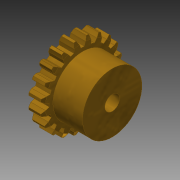
# Autodesk Inventor part: Zahnrad Messing z20
Saved by Autodesk Inventor 2019.4 (Build 234330000, 330)
## iProperties
Category: PARTsolutions
Company: MAEDLER
Created: 2018-08-20
Part Number: Zahnrad Messing z20
Material: Messing, weicher Gelbton, geschweißt
Catalog Web Link: www.cadenas.de
Description: Stzr Messing Ms58-Spur Gears, Brass, Helical Tooth Right Hand, with one-sided hub
Vendor: MAEDLER
Document SubType Name: Modeling
Designer: psadmin
Manufacturer: MAEDLER
Mass: 2.8 g
Surface Area: 3.98913 cm^2
Volume: 0.336189 cm^3
Density: 8.32866 g/cm^3
Appearance: Schweißnaht - Messing
PSOL_IDENT_0: {$CADENAS_DATA\23d-libs\maedler\antriebselemente\stirnzahnraeder\stirnzahnraeder_messing\stzr_messin
PSOL_IDENT_1: g_ms58.prj},204 {VTYP=3D},{NB=Stzr Messing Ms58 26102000},{LINA=Stzr Messing Ms58 26102000},{NN=Stzr
PSOL_IDENT_2: Messing Ms58},{DATE=03.08.2018 09:08:56},{GEOMDATE=26.07.2018 09:15:44},{VERSION=},{LINEID=270},{WB
PSOL_IDENT_3: VAR=},{WBNUMERIC=}  {NB=Stzr Messing Ms58 26102000},{LINA=Stzr Messing Ms58 26102000},{KT=DUMMY},{AR
PSOL_IDENT_4: TNR=26102000},{WST=Messing (Ms58)},{M=0.5},{Z=20},{PDF=PDF Katalogseite},{B1=2.0},{DA=11.00},{D=10.0
PSOL_IDENT_5: 0},{NL=4},{ND=8},{B=2.00},{MD=1.2},{GEW=2.800}
NN: Stzr Messing Ms58
NT: Spur Gears, Brass, Helical Tooth Right Hand, with one-sided hub
NB: Stzr Messing Ms58 26102000
NBSYN: Stzr Messing Ms58 $ARTNR.
LINA: Stzr Messing Ms58 26102000
ARTNR: 26102000
WST: Messing (Ms58)
M: 0.5
Z: 20
PDF: PDF Katalogseite
B1: 2
DA: 11
D: 10
NL: 4
ND: 8
B: 2
MD: 1.2
GEW: 2.8
SUPPLIER: MAEDLER
ARTICLENO: Stzr Messing Ms58 26102000
BOMINFO: Stzr Messing Ms58 26102000
CREATOR: CADENAS GmbH
Title: Stzr Messing Ms58 26102000
Author: Cadenas PARTsolutions
Comments: Spur Gears, Brass, Helical Tooth Right Hand, with one-sided hub
Autodesk Inventor part; units mm, degrees
ref_plane "YZ Plane" through (0, 0, 0) normal (1, 0, 0) x (0, 1, 0)
ref_plane "XZ Plane" through (0, 0, 0) normal (0, 1, 0) x (-1, 0, 0)
ref_plane "XY Plane" through (0, 0, 0) normal (0, 0, 1) x (1, 0, 0)
sketch "Skizze_1" plane through (0, 0, 0) normal (0, 0, 1) x (1, 0, 0)
  line L0 (6, 0) -> (0, 0)
  line L1 (0, 1) -> (6, 1)
  line L2 (6, 1) -> (6, 4)
  line L3 (6, 4) -> (2, 4)
  line L4 (2, 4) -> (2, 5)
  line L5 (2, 5) -> (1, 7.7475)
  line L6 (1, 7.7475) -> (0, 5)
  line L7 (0, 5) -> (0, 1)
  constraints: 16 end point
revolve "Revolution1" add sketch "Skizze_1" angle 360 about axis through (6, 0, 0) along (1, 0, 0)
sketch "Skizze_2" plane through (2, 0, 0) normal (1, 0, 0) x (0, 0, -1)
  circle A0 centre (0, 0) radius 16.5
  arc A1 (-5.4559, -0.6954) -> (-5.4037, -1.0246) centre (0, 0) ccw
  line L0 (-5.4037, -1.0246) -> (-4.8668, -1.1465)
  line L1 (-4.8668, -1.1465) -> (-4.3467, -1.1647)
  arc A2 (-4.3467, -1.1647) -> (-4.2011, -1.6127) centre (0, 0) ccw
  line L2 (-4.2011, -1.6127) -> (-4.6112, -1.9331)
  line L3 (-4.6112, -1.9331) -> (-4.974, -2.3473)
  arc A3 (-4.974, -2.3473) -> (-4.8226, -2.6443) centre (0, 0) ccw
  line L4 (-4.8226, -2.6443) -> (-4.2743, -2.5943)
  line L5 (-4.2743, -2.5943) -> (-3.774, -2.4509)
  arc A4 (-3.774, -2.4509) -> (-3.4972, -2.8319) centre (0, 0) ccw
  line L6 (-3.4972, -2.8319) -> (-3.7882, -3.2634)
  line L7 (-3.7882, -3.2634) -> (-4.0052, -3.7695)
  arc A5 (-4.0052, -3.7695) -> (-3.7695, -4.0052) centre (0, 0) ccw
  line L8 (-3.7695, -4.0052) -> (-3.2634, -3.7882)
  line L9 (-3.2634, -3.7882) -> (-2.8319, -3.4972)
  arc A6 (-2.8319, -3.4972) -> (-2.4509, -3.774) centre (0, 0) ccw
  line L10 (-2.4509, -3.774) -> (-2.5943, -4.2743)
  line L11 (-2.5943, -4.2743) -> (-2.6443, -4.8226)
  arc A7 (-2.6443, -4.8226) -> (-2.3473, -4.974) centre (0, 0) ccw
  line L12 (-2.3473, -4.974) -> (-1.9331, -4.6112)
  line L13 (-1.9331, -4.6112) -> (-1.6127, -4.2011)
  arc A8 (-1.6127, -4.2011) -> (-1.1647, -4.3467) centre (0, 0) ccw
  line L14 (-1.1647, -4.3467) -> (-1.1465, -4.8668)
  line L15 (-1.1465, -4.8668) -> (-1.0246, -5.4037)
  arc A9 (-1.0246, -5.4037) -> (-0.6954, -5.4559) centre (0, 0) ccw
  line L16 (-0.6954, -5.4559) -> (-0.4135, -4.9829)
  line L17 (-0.4135, -4.9829) -> (-0.2355, -4.4938)
  arc A10 (-0.2355, -4.4938) -> (0.2355, -4.4938) centre (0, 0) ccw
  line L18 (0.2355, -4.4938) -> (0.4135, -4.9829)
  line L19 (0.4135, -4.9829) -> (0.6954, -5.4559)
  arc A11 (0.6954, -5.4559) -> (1.0246, -5.4037) centre (0, 0) ccw
  line L20 (1.0246, -5.4037) -> (1.1465, -4.8668)
  line L21 (1.1465, -4.8668) -> (1.1647, -4.3467)
  arc A12 (1.1647, -4.3467) -> (1.6127, -4.2011) centre (0, 0) ccw
  line L22 (1.6127, -4.2011) -> (1.9331, -4.6112)
  line L23 (1.9331, -4.6112) -> (2.3473, -4.974)
  arc A13 (2.3473, -4.974) -> (2.6443, -4.8226) centre (0, 0) ccw
  line L24 (2.6443, -4.8226) -> (2.5943, -4.2743)
  line L25 (2.5943, -4.2743) -> (2.4509, -3.774)
  arc A14 (2.4509, -3.774) -> (2.8319, -3.4972) centre (0, 0) ccw
  line L26 (2.8319, -3.4972) -> (3.2634, -3.7882)
  line L27 (3.2634, -3.7882) -> (3.7695, -4.0052)
  arc A15 (3.7695, -4.0052) -> (4.0052, -3.7695) centre (0, 0) ccw
  line L28 (4.0052, -3.7695) -> (3.7882, -3.2634)
  line L29 (3.7882, -3.2634) -> (3.4972, -2.8319)
  arc A16 (3.4972, -2.8319) -> (3.774, -2.4509) centre (0, 0) ccw
  line L30 (3.774, -2.4509) -> (4.2743, -2.5943)
  line L31 (4.2743, -2.5943) -> (4.8226, -2.6443)
  arc A17 (4.8226, -2.6443) -> (4.974, -2.3473) centre (0, 0) ccw
  line L32 (4.974, -2.3473) -> (4.6112, -1.9331)
  line L33 (4.6112, -1.9331) -> (4.2011, -1.6127)
  arc A18 (4.2011, -1.6127) -> (4.3467, -1.1647) centre (0, 0) ccw
  line L34 (4.3467, -1.1647) -> (4.8668, -1.1465)
  line L35 (4.8668, -1.1465) -> (5.4037, -1.0246)
  arc A19 (5.4037, -1.0246) -> (5.4559, -0.6954) centre (0, 0) ccw
  line L36 (5.4559, -0.6954) -> (4.9829, -0.4135)
  line L37 (4.9829, -0.4135) -> (4.4938, -0.2355)
  arc A20 (4.4938, -0.2355) -> (4.4938, 0.2355) centre (0, 0) ccw
  line L38 (4.4938, 0.2355) -> (4.9829, 0.4135)
  line L39 (4.9829, 0.4135) -> (5.4559, 0.6954)
  arc A21 (5.4559, 0.6954) -> (5.4037, 1.0246) centre (0, 0) ccw
  line L40 (5.4037, 1.0246) -> (4.8668, 1.1465)
  line L41 (4.8668, 1.1465) -> (4.3467, 1.1647)
  arc A22 (4.3467, 1.1647) -> (4.2011, 1.6127) centre (0, 0) ccw
  line L42 (4.2011, 1.6127) -> (4.6112, 1.9331)
  line L43 (4.6112, 1.9331) -> (4.974, 2.3473)
  arc A23 (4.974, 2.3473) -> (4.8226, 2.6443) centre (0, 0) ccw
  line L44 (4.8226, 2.6443) -> (4.2743, 2.5943)
  line L45 (4.2743, 2.5943) -> (3.774, 2.4509)
  arc A24 (3.774, 2.4509) -> (3.4972, 2.8319) centre (0, 0) ccw
  line L46 (3.4972, 2.8319) -> (3.7882, 3.2634)
  line L47 (3.7882, 3.2634) -> (4.0052, 3.7695)
  arc A25 (4.0052, 3.7695) -> (3.7695, 4.0052) centre (0, 0) ccw
  line L48 (3.7695, 4.0052) -> (3.2634, 3.7882)
  line L49 (3.2634, 3.7882) -> (2.8319, 3.4972)
  arc A26 (2.8319, 3.4972) -> (2.4509, 3.774) centre (0, 0) ccw
  line L50 (2.4509, 3.774) -> (2.5943, 4.2743)
  line L51 (2.5943, 4.2743) -> (2.6443, 4.8226)
  arc A27 (2.6443, 4.8226) -> (2.3473, 4.974) centre (0, 0) ccw
  line L52 (2.3473, 4.974) -> (1.9331, 4.6112)
  line L53 (1.9331, 4.6112) -> (1.6127, 4.2011)
  arc A28 (1.6127, 4.2011) -> (1.1647, 4.3467) centre (0, 0) ccw
  line L54 (1.1647, 4.3467) -> (1.1465, 4.8668)
  line L55 (1.1465, 4.8668) -> (1.0246, 5.4037)
  arc A29 (1.0246, 5.4037) -> (0.6954, 5.4559) centre (0, 0) ccw
  line L56 (0.6954, 5.4559) -> (0.4135, 4.9829)
  line L57 (0.4135, 4.9829) -> (0.2355, 4.4938)
  arc A30 (0.2355, 4.4938) -> (-0.2355, 4.4938) centre (0, 0) ccw
  line L58 (-0.2355, 4.4938) -> (-0.4135, 4.9829)
  line L59 (-0.4135, 4.9829) -> (-0.6954, 5.4559)
  arc A31 (-0.6954, 5.4559) -> (-1.0246, 5.4037) centre (0, 0) ccw
  line L60 (-1.0246, 5.4037) -> (-1.1465, 4.8668)
  line L61 (-1.1465, 4.8668) -> (-1.1647, 4.3467)
  arc A32 (-1.1647, 4.3467) -> (-1.6127, 4.2011) centre (0, 0) ccw
  line L62 (-1.6127, 4.2011) -> (-1.9331, 4.6112)
  line L63 (-1.9331, 4.6112) -> (-2.3473, 4.974)
  arc A33 (-2.3473, 4.974) -> (-2.6443, 4.8226) centre (0, 0) ccw
  line L64 (-2.6443, 4.8226) -> (-2.5943, 4.2743)
  line L65 (-2.5943, 4.2743) -> (-2.4509, 3.774)
  arc A34 (-2.4509, 3.774) -> (-2.8319, 3.4972) centre (0, 0) ccw
  line L66 (-2.8319, 3.4972) -> (-3.2634, 3.7882)
  line L67 (-3.2634, 3.7882) -> (-3.7695, 4.0052)
  arc A35 (-3.7695, 4.0052) -> (-4.0052, 3.7695) centre (0, 0) ccw
  line L68 (-4.0052, 3.7695) -> (-3.7882, 3.2634)
  line L69 (-3.7882, 3.2634) -> (-3.4972, 2.8319)
  arc A36 (-3.4972, 2.8319) -> (-3.774, 2.4509) centre (0, 0) ccw
  line L70 (-3.774, 2.4509) -> (-4.2743, 2.5943)
  line L71 (-4.2743, 2.5943) -> (-4.8226, 2.6443)
  arc A37 (-4.8226, 2.6443) -> (-4.974, 2.3473) centre (0, 0) ccw
  line L72 (-4.974, 2.3473) -> (-4.6112, 1.9331)
  line L73 (-4.6112, 1.9331) -> (-4.2011, 1.6127)
  arc A38 (-4.2011, 1.6127) -> (-4.3467, 1.1647) centre (0, 0) ccw
  line L74 (-4.3467, 1.1647) -> (-4.8668, 1.1465)
  line L75 (-4.8668, 1.1465) -> (-5.4037, 1.0246)
  arc A39 (-5.4037, 1.0246) -> (-5.4559, 0.6954) centre (0, 0) ccw
  line L76 (-5.4559, 0.6954) -> (-4.9829, 0.4135)
  line L77 (-4.9829, 0.4135) -> (-4.4938, 0.2355)
  arc A40 (-4.4938, 0.2355) -> (-4.4938, -0.2355) centre (0, 0) ccw
  line L78 (-4.4938, -0.2355) -> (-4.9829, -0.4135)
  line L79 (-4.9829, -0.4135) -> (-5.4559, -0.6954)
  constraints: 160 end point, 80 point on circle, 41 centre point
extrude "Extrusion1" cut sketch "Skizze_2" along normal mid plane 12
sketch "Skizze3" plane through (6, 0, 0) normal (1, 0, 0) x (0, 0, -1)
  circle A0 centre (0, 0) radius 4 projected
extrude "Extrusion2" [suppressed]
sketch "Skizze4" plane through (0, 0, 0) normal (-1, 0, 0) x (0, 0, 1)
  point P0 (0, 0)
  point P1 (0, 0)
  constraints: 1 coincident
hole "Bohrung1" [suppressed]
body "Solid1"
